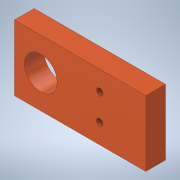
# Autodesk Inventor part: Part4
Saved by Autodesk Inventor 2020 (Build 240168000, 168)
## iProperties
Created: 2020-03-11
Part Number: Part4
Material: Generic
Document SubType Name: Modeling
Designer: tor16003
Density: 1 g/cm^3
Appearance: Suave - Naranja claro
Author: tor16003
Autodesk Inventor part; units mm, degrees
ref_plane "YZ Plane" through (0, 0, 0) normal (1, 0, 0) x (0, 1, 0)
ref_plane "XZ Plane" through (0, 0, 0) normal (0, 1, 0) x (-1, 0, 0)
ref_plane "XY Plane" through (0, 0, 0) normal (0, 0, 1) x (1, 0, 0)
sketch "Sketch1" plane through (0, 0, 0) normal (0, 0, 1) x (1, 0, 0)
  line L0 (0, 0) -> (20, 0)
  line L1 (20, 0) -> (20, 10)
  line L2 (20, 10) -> (0, 10)
  line L3 (0, 10) -> (0, 0)
  circle A0 centre (4, 5) radius 2.5
  circle A1 centre (13, 3) radius 0.5
  circle A2 centre (13, 7) radius 0.5
  point P0 (0, 5)
  dimension "d0" = 20
  dimension "d1" = 10
  dimension "d3" = 5
  dimension "d4" = 4
  dimension "d7" = 1
  dimension "d8" = 1
  dimension "d9" = 4
  dimension "d10" = 3
  dimension "d11" = 13
  constraints: 8 end point, 3 centre point, 2 parallel, 1 horizontal, 1 horizontal alignment, 1 midpoint, 1 perpendicular, 1 vertical alignment
  measures "d0" distance of L2.end L1.end
  measures "d1" distance of L1.end L0.end
  measures "d3" diameter of A0
  measures "d4" distance from line of L3 A0.centre
  measures "d7" diameter of A1
  measures "d8" diameter of A2
  measures "d9" distance of A2.centre A1.centre
  measures "d10" distance from line of L2 A2.centre
  measures "d11" distance from line of L3 A1.centre
extrude "Extrusión1" add sketch "Sketch1" along normal blind 3
